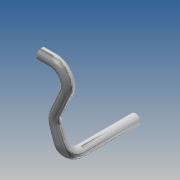
# Autodesk Inventor part: exhaust header right pipe 3
Saved by Autodesk Inventor 2013 (Build 170138000, 138)
## iProperties
Created: 2013-02-09
Part Number: exhaust header right pipe 3
Material: Steel
Document SubType Name: Modeling
Designer: zhaphod
Density: 1 g/cm^3
Author: zhaphod
Autodesk Inventor part; units mm, degrees
sketch "Sketch1" plane through (0, 0, 0) normal (1, 0, 0) x (0, 1, 0)
  line L0 (0, 0) -> (0, -200)
  line L1 (0, -200) -> (0, -332.225)
  line L2 (0, -332.225) -> (291.85, -332.225)
  line L3 (0, 0) -> (0, -144.4625) construction
  line L4 (0, -144.4625) -> (0, -52.775) construction
  line L5 (0, -52.775) -> (0, -97.225) construction
  line L6 (0, -97.225) -> (291.85, -97.225) construction
  dimension "d0" = 332.225
  dimension "d1" = 0
  dimension "d4" = 200
  dimension "d5" = 291.85
  dimension "d6" = 144.4625
  dimension "d7" = 97.225
  dimension "d8" = 52.775
  constraints: 14 end point, 3 vertical alignment, 2 perpendicular, 1 horizontal, 1 vertical
  measures "d0" distance from line of L2 L0.start
  measures "d1" horizontal distance of L0.end L0.start
  measures "d4" distance of L0.end L0.start
  measures "d5" horizontal distance of L0.start L2.end
  measures "d6" distance of L0.start L3.end
  measures "d7" distance from line of L6 L0.start
  measures "d8" distance of L4.end L0.start
ref_plane "Work Plane1" through (144.4625, 0, 0) normal (1, 0, 0) x (0, 1, 0)
ref_plane "Work Plane2" through (52.775, 0, 0) normal (1, 0, 0) x (0, 1, 0)
ref_plane "Work Plane3" through (97.225, 0, 0) normal (1, 0, 0) x (0, 1, 0)
sketch "Sketch2" plane through (144.4625, 0, 0) normal (1, 0, 0) x (0, 1, 0)
  point P0 (0, 0)
  point P1 (0, 0)
sketch "Sketch3" plane through (52.775, 0, 0) normal (1, 0, 0) x (0, 1, 0)
  point P0 (0, 0)
  point P1 (0, -200)
  point P2 (0, -332.225)
sketch "Sketch4" plane through (97.225, 0, 0) normal (1, 0, 0) x (0, 1, 0)
  point P0 (0, 0)
  point P1 (291.85, -332.225)
  point P2 (0, -332.225)
sketch "Sketch5" plane through (0, 0, 0) normal (1, 0, 0) x (0, 1, 0)
  circle A0 centre (0, 0) radius 20.6375
  circle A1 centre (0, 0) radius 19.0375
  dimension "d15" = 1.6
  dimension "d17" = 41.275
  constraints: 2 centre point, 2 coincident
  measures "d15" radial gap between concentric circles of A0 A1
  measures "d17" diameter of A0
sketch3d "3D Sketch1"
  line L0 (0, 0, 0) -> (47.9711, 0, 0)
  arc A0 (47.9711, 0, 0) -> (104.2514, 0, -87.7135) centre (47.9711, 0, -61.9125) ccw
  line L1 (104.2514, 0, -87.7135) -> (62.9928, 0, -177.7116)
  arc A1 (62.9928, 0, -177.7116) -> (60.5878, 0, -223.2408) centre (119.2731, 0, -203.5126) ccw
  line L2 (60.5878, 0, -223.2408) -> (77.4968, 0, -273.5398)
  arc A2 (77.4968, 0, -273.5398) -> (97.225, 61.9125, -332.225) centre (77.4968, 61.9125, -273.5398) ccw
  line L3 (97.225, 61.9125, -332.225) -> (97.225, 291.85, -332.225)
  dimension "d14" = 61.9125
  dimension "d12" = 61.9125
  dimension "d13" = 61.9125
  constraints: 4 vertical
sweep "Sweep1" add profiles "Sketch5" path "3D Sketch1"
equation "\"d14\" = d12"
equation "\"d13\" = d12"
equation "\"d9\" = d6"
equation "\"d10\" = d8"
equation "\"d11\" = d7"
body "Solid1"
